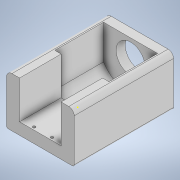
# Autodesk Inventor part: Motor_Mount
Saved by Autodesk Inventor 2022 (Build 260153000, 153)
## iProperties
Created: 2022-01-23
Part Number: Motor_Mount
Material: Generic
Document SubType Name: Modeling
Designer: Mlees
Density: 1 g/cm^3
Appearance: Default
Author: Mlees
Autodesk Inventor part; units mm, degrees
ref_plane "YZ Plane" through (0, 0, 0) normal (1, 0, 0) x (0, 1, 0)
ref_plane "XZ Plane" through (0, 0, 0) normal (0, 1, 0) x (-1, 0, 0)
ref_plane "XY Plane" through (0, 0, 0) normal (0, 0, 1) x (1, 0, 0)
sketch "Sketch1" plane through (0, 0, 0) normal (0, 1, 0) x (-1, 0, 0)
  line L0 (0, 0) -> (75, 0)
  line L1 (75, 0) -> (75, -91)
  line L2 (75, -91) -> (0, -91)
  line L3 (0, -91) -> (0, 0)
  dimension "d0" = 75
  dimension "d1" = 91
  constraints: 8 end point, 2 parallel, 1 horizontal, 1 perpendicular
  measures "d0" distance of L1.end L2.end
  measures "d1" distance of L0.end L1.end
extrude "Extrusion1" add sketch "Sketch1" along normal blind 5
sketch "Sketch2" plane through (0, 5, 0) normal (0, 1, 0) x (1, 0, 0)
  line L0 (-14.5, 42) -> (0, 42)
  line L1 (0, 0) -> (0, 91) projected
  line L2 (0, 42) -> (0, 0)
  line L3 (0, 0) -> (-14.5, 0)
  line L4 (0, 91) -> (-75, 91) projected
  line L5 (-60.5, 42) -> (-75, 42)
  line L6 (-75, 42) -> (-75, 0)
  line L7 (-75, 0) -> (-60.5, 0)
  line L8 (-60.5, 42) -> (-14.5, 42)
  line L9 (-14.5, 0) -> (-60.5, 0)
  line L10 (-75, 0) -> (0, 0) projected
  constraints: 16 end point, 2 collinear, 2 perpendicular, 1 point on line
extrude "Extrusion2" add sketch "Sketch2" along normal blind 8
sketch "Sketch3" plane through (0, 0, -91) normal (0, 0, -1) x (-1, 0, 0)
  line L0 (0, 5) -> (75, 5) projected
  line L1 (75, 0) -> (0, 0) projected
  line L2 (0, 5) -> (75, 5)
  line L3 (75, 5) -> (75, 0)
  line L4 (75, 0) -> (0, 0)
  line L5 (0, 0) -> (0, 5)
  constraints: 8 end point, 2 parallel, 1 horizontal, 1 perpendicular
extrude "Extrusion3" add sketch "Sketch3" along normal blind 15
sketch "Sketch4" plane through (0, 13, 0) normal (0, 1, 0) x (1, 0, 0)
  line L0 (-14.5, 0) -> (-14.5, 42)
  line L1 (0, 42) -> (-75, 42) projected
  line L2 (-60.5, 0) -> (-60.5, 42)
  line L3 (-75, 0) -> (0, 0) projected
  line L4 (0, 0) -> (-14.5, 0)
  line L5 (-14.5, 0) -> (-14.5, 42)
  line L6 (-14.5, 42) -> (0, 42)
  line L7 (0, 42) -> (0, 0)
  line L8 (-60.5, 42) -> (-75, 42)
  line L9 (-75, 42) -> (-75, 0)
  line L10 (-75, 0) -> (-60.5, 0)
  line L11 (-60.5, 0) -> (-60.5, 42)
  constraints: 20 end point, 4 parallel, 2 horizontal, 2 perpendicular, 1 point on line
extrude "Extrusion4" add sketch "Sketch4" along normal blind 42 contours L0 L1 L7 L3 | L3 L9 L1 L2
sketch "Sketch5" plane through (0, 0, -106) normal (0, 0, -1) x (-1, 0, 0)
  line L0 (75, 5) -> (0, 5) projected
  line L1 (37.5, 5) -> (19.472, 5)
  line L2 (19.472, 5) -> (55.528, 5)
  line L3 (37.5, 5) -> (37.5, 35)
  line L4 (75, 0) -> (75, 55) projected
  line L5 (0, 5) -> (0, 55) projected
  line L6 (37.5, 35) -> (7.5, 35)
  line L7 (67.5, 35) -> (67.5, 16.972)
  line L8 (67.5, 35) -> (67.5, 53.028)
  arc A0 (55.528, 5) -> (67.5, 16.972) centre (37.5001, 34.9999) ccw
  line L9 (7.5, 35) -> (7.5, 53.028)
  line L10 (7.5, 35) -> (7.5, 16.9723)
  arc A1 (7.5, 16.9723) -> (19.472, 5) centre (37.5014, 35.001) ccw
  line L11 (67.5, 53.028) -> (75, 53.028)
  line L12 (75, 0) -> (0, 0) projected
  line L13 (75, 53.028) -> (75, 0)
  line L14 (75, 0) -> (0, 0)
  line L15 (0, 0) -> (0, 53.028)
  line L16 (7.5, 53.028) -> (0, 53.028)
  dimension "d18" = 18.028
  dimension "d19" = 36.056
  dimension "d20" = 30
  dimension "d21" = 30
  dimension "d22" = 30
  dimension "d23" = 18.028
  dimension "d24" = 18.028
  dimension "d25" = 35
  constraints: 26 end point, 6 vertical, 5 point on line, 4 point on circle, 3 perpendicular, 2 centre point, 1 horizontal, 1 midpoint
  measures "d18" distance of L1.start L1.end
  measures "d19" distance of L1.end L2.end
  measures "d20" distance of L1.start L3.end
  measures "d21" distance of L3.end L7.start
  measures "d22" distance of L3.end L6.end
  measures "d23" distance of L7.start L7.end
  measures "d24" distance of L7.start L8.end
  measures "d25" radius of A0
extrude "Extrusion5" add sketch "Sketch5" against normal up to surface (64 mm away) contours L0 A0 L7 L8 L11 L4 | L0 L5 L16 L9 L10 A1
sketch "Sketch6" plane through (-75, 0, 0) normal (0, 0, 1) x (1, 0, 0)
  line L0 (0, 0) -> (0, 55) projected
  line L1 (75, 0) -> (0, 0) projected
  line L2 (0, 55) -> (0, 0)
  line L3 (0, 0) -> (75, 0)
  line L4 (75, 53.028) -> (75, 55) projected
  line L5 (75, 0) -> (75, 55)
  line L6 (75, 55) -> (60.5, 55) projected
  line L7 (75, 55) -> (60.5, 55)
  line L8 (60.5, 13) -> (60.5, 55) projected
  line L9 (60.5, 55) -> (60.5, 13)
  line L10 (60.5, 13) -> (14.5, 13) projected
  line L11 (60.5, 13) -> (14.5, 13)
  line L12 (14.5, 13) -> (14.5, 55) projected
  line L13 (14.5, 13) -> (14.5, 55)
  line L14 (14.5, 55) -> (0, 55)
  constraints: 16 end point, 6 perpendicular, 2 collinear
extrude "Extrusion6" add sketch "Sketch6" along normal blind 4
sketch "Sketch8" plane through (0, 0, 0) normal (0, -1, 0) x (1, 0, 0)
  line L0 (-14.5, 4) -> (-60.5, 4) projected
  point P0 (0, 0)
  point P1 (-27.5, 1)
  point P2 (-47.5, 1)
hole "Hole2" at (-27.5, 0, 1) at (-47.5, 0, 1) direction (0, 1, 0) diameter 3 end through all counterbore diameter 5 counterbore depth 2
sketch "Sketch9" plane through (0, 55, 0) normal (0, 1, 0) x (1, 0, 0)
  point P0 (0, 0)
sketch "Sketch10" plane through (0, 5, 0) normal (0, 1, 0) x (1, 0, 0)
  line L0 (-67.5, 106) -> (-67.5, 42) projected
  line L1 (-7.5, 106) -> (-67.5, 106)
  line L2 (-67.5, 106) -> (-67.5, 96)
  line L3 (-67.5, 96) -> (-7.5, 96)
  line L4 (-7.5, 106) -> (-7.5, 42) projected
  line L5 (-7.5, 96) -> (-7.5, 106)
  point P0 (0, 0)
  dimension "d50" = 10
  constraints: 8 end point, 4 perpendicular, 1 point on line
  measures "d50" distance of L0.start L2.end
extrude "Extrusion7" add sketch "Sketch10" along normal up to surface (48.028 mm away)
sketch "Sketch11" plane through (0, 0, -106) normal (0, 0, -1) x (-1, 0, 0)
  line L0 (55.528, 5) -> (19.472, 5) projected
  circle A0 centre (37.5, 35) radius 16.5
  point P0 (0, 0)
  dimension "d56" = 33
  constraints: 1 centre point
  measures "d56" diameter of A0
extrude "Extrusion8" cut sketch "Sketch11" against normal through all
sketch "Sketch12" plane through (-75, 53.028, -106) normal (0, 1, 0) x (1, 0, 0)
  line L0 (75, -64) -> (67.5, -64) projected
  line L1 (75, 0) -> (75, -64) projected
  line L2 (75, -64) -> (75, 0)
  line L3 (75, 0) -> (0, 0) projected
  line L4 (75, 0) -> (0, 0)
  line L5 (7.5, -64) -> (0, -64) projected
  line L6 (0, 0) -> (0, -64)
  line L7 (7.5, -10) -> (7.5, -64) projected
  line L8 (0, -64) -> (7.5, -64)
  line L9 (7.5, -64) -> (7.5, -10)
  line L10 (67.5, -10) -> (7.5, -10) projected
  line L11 (7.5, -10) -> (67.5, -10)
  line L12 (67.5, -10) -> (67.5, -64) projected
  line L13 (67.5, -10) -> (67.5, -64)
  line L14 (67.5, -64) -> (75, -64)
  point P0 (75, -106)
  constraints: 16 end point, 5 perpendicular, 2 collinear, 1 vertical
extrude "Extrusion9" add sketch "Sketch12" along normal up to surface (1.972 mm away)
fillet "Fillet2" radius 2 2 edges at (0, 0, -51) (-75, 0, -51)
fillet "Fillet3" radius 6 2 edges at (0, 55, -51) (-75, 55, -51)
sketch "Sketch13" plane through (0, 0, 0) normal (0, -1, 0) x (1, 0, 0)
  line L0 (-2, 4) -> (-2, -106) projected
  line L1 (-73, -106) -> (-73, 4) projected
  circle A0 centre (-27.5, -31) radius 1.5
  circle A1 centre (-47.5, -31) radius 1.5
  circle A2 centre (-47.5, -71) radius 1.5
  circle A3 centre (-27.5, -71) radius 1.5
  point P0 (0, 0)
  dimension "d68" = 3
  constraints: 4 centre point
  measures "d68" diameter of A0
extrude "Extrusion10" cut sketch "Sketch13" against normal blind 10
sketch "Sketch14" plane through (0, 0, -106) normal (0, 0, -1) x (-1, 0, 0)
  circle A0 centre (37.5, 35) radius 16.5 projected
  circle A1 centre (37.5, 35) radius 16
  point P0 (0, 0)
  dimension "d71" = 32
  constraints: 1 centre point, 1 coincident
  measures "d71" diameter of A1
extrude "Extrusion11" add sketch "Sketch14" against normal up to surface (10 mm away)
body "Solid1"
